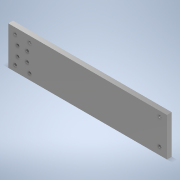
# Autodesk Inventor part: Corner Stands
Saved by Autodesk Inventor 2020 (Build 240168000, 168)
## iProperties
Created: 2020-03-17
Part Number: Corner Stands
Material: Generic
Document SubType Name: Modeling
Designer: DasNick
Density: 1 g/cm^3
Appearance: Anodized - Light Gray
Author: DasNick
Autodesk Inventor part; units mm, degrees
ref_plane "YZ Plane" through (0, 0, 0) normal (1, 0, 0) x (0, 1, 0)
ref_plane "XZ Plane" through (0, 0, 0) normal (0, 1, 0) x (-1, 0, 0)
ref_plane "XY Plane" through (0, 0, 0) normal (0, 0, 1) x (1, 0, 0)
sketch "Sketch1" plane through (0, 0, 0) normal (0, 0, 1) x (1, 0, 0)
  line L0 (246.3741, 31.7234) -> (246.3741, -882.6766) construction
  line L1 (234.1821, 31.7234) -> (231.3881, 31.7234) construction
  line L2 (223.2601, 31.7234) -> (220.4661, 31.7234) construction
  line L3 (199.5111, 31.7234) -> (196.0821, 31.7234) construction
  line L4 (182.3661, 31.7234) -> (178.9371, 31.7234) construction
  line L5 (246.3741, 31.7234) -> (170.1741, 31.7234)
  line L6 (170.1741, 31.7234) -> (170.1741, -69.8766)
  line L7 (170.1741, -69.8766) -> (246.3741, -69.8766)
  line L8 (246.3741, -69.8766) -> (246.3741, 31.7234)
  circle A0 centre (227.3241, 15.8484) radius 3.9688
  line L9 (208.2741, -69.8766) -> (208.2741, 31.7234) construction
  line L10 (246.3741, -19.0766) -> (170.1741, -19.0766) construction
  circle A1 centre (227.3241, -54.0016) radius 3.9688
  circle A2 centre (189.2241, 15.8484) radius 3.9688
  circle A3 centre (189.2241, -54.0016) radius 3.9688
  point P0 (0, 0)
  dimension "d0" = 76.2
  dimension "d1" = 101.6
  dimension "d2" = 7.9375
  dimension "d3" = 15.875
  dimension "d4" = 19.05
  constraints: 12 end point, 4 centre point, 4 midpoint, 3 symmetric about line, 2 parallel, 1 horizontal, 1 perpendicular, 3 other
  measures "d0" distance of L7.end L6.end
  measures "d1" distance of L6.end L5.end
  measures "d2" diameter of A0
  measures "d3" distance from line of L5 A0.centre
  measures "d4" distance from line of L0 A0.centre
extrude "Extrusion1" add sketch "Sketch1" along normal blind 12.7
sketch "Sketch3" plane through (0, 0, 0) normal (0, 0, -1) x (-1, 0, 0)
  line L0 (-186.0491, -41.3016) -> (-230.4991, -41.3016)
  line L1 (-230.4991, -41.3016) -> (-230.4991, 3.1484)
  line L2 (-230.4991, 3.1484) -> (-186.0491, 3.1484)
  line L3 (-186.0491, 3.1484) -> (-186.0491, -41.3016)
  line L4 (-170.1741, -69.8766) -> (-246.3741, -69.8766) projected
  line L5 (-170.1741, 31.7234) -> (-170.1741, -69.8766) projected
  line L6 (-246.3741, 31.7234) -> (-170.1741, 31.7234) projected
  circle A0 centre (-195.5741, -6.3766) radius 6.35
  circle A1 centre (-195.5741, -31.7766) radius 6.35
  circle A2 centre (-220.9741, -6.3766) radius 6.35
  circle A3 centre (-220.9741, -31.7766) radius 6.35
  point P0 (0, 0)
  dimension "d16" = 44.45
  dimension "d17" = 44.45
  dimension "d18" = 28.575
  dimension "d19" = 15.875
  dimension "d23" = 12.7
  dimension "d24" = 9.525
  dimension "d25" = 9.525
  dimension "d28" = 25.4
  dimension "d31" = 25.4
  constraints: 8 end point, 4 centre point, 2 horizontal, 2 parallel, 1 perpendicular, 1 vertical, 7 other
  measures "d16" distance of L0.end L1.end
  measures "d17" distance of L0.start L0.end
  measures "d18" distance between parallel lines of L4 L0
  measures "d19" distance between parallel lines of L5 L3
  measures "d23" diameter of A0
  measures "d24" distance from line of L2 A0.centre
  measures "d25" distance from line of L3 A0.centre
  measures "d28" distance of A0.centre A1.centre
  measures "d31" distance of A0.centre A2.centre
extrude "Extrusion3" cut sketch "Sketch3" against normal blind 7.9375 contours A0 | A1 | A2 | A3
sketch "Sketch4" plane through (195.5741, -6.3766, 7.9375) normal (0, 0, -1) x (-1, 0, 0)
  circle A0 centre (0, 0) radius 6.35 projected
  circle A1 centre (0, -25.4) radius 6.35 projected
  circle A2 centre (-25.4, 0) radius 6.35 projected
  circle A3 centre (-25.4, -25.4) radius 6.35 projected
  circle A4 centre (0, 0) radius 3.9688
  line L0 (0, 0) -> (0, -11.1628) construction
  line L1 (0, 0) -> (-15.7699, 0) construction
  circle A5 centre (0, -25.4) radius 3.9688
  circle A6 centre (-25.4, 0) radius 3.9688
  circle A7 centre (-25.4, -25.4) radius 3.9688
  point P0 (195.5741, 6.3766)
  dimension "d36" = 7.9375
  dimension "d37" = 7.9375
  dimension "d38" = 7.9375
  dimension "d39" = 7.9375
  constraints: 4 centre point, 4 coincident, 4 end point, 1 horizontal, 1 vertical
  measures "d36" diameter of A4
  measures "d37" diameter of A5
  measures "d38" diameter of A6
  measures "d39" diameter of A7
extrude "Extrusion4" cut sketch "Sketch4" against normal blind 7.9375 contours A4 | A5 | A6 | A7
sketch "Sketch5" plane through (0, 0, 12.7) normal (0, 0, 1) x (1, 0, 0)
  line L0 (589.2741, -69.8766) -> (589.2741, 844.5234)
  line L1 (246.3741, -69.8766) -> (589.2741, -69.8766)
  line L2 (246.3741, 31.7234) -> (170.1741, 31.7234) projected
  line L3 (246.3741, 31.7234) -> (589.2741, 31.7234)
  line L4 (376.7143, 0.5706) -> (376.7143, -56.5544)
  line L5 (376.7143, 18.2956) -> (376.7143, 9.7706)
  line L6 (376.7143, 18.2956) -> (376.7143, 23.7956)
  line L7 (376.7143, -62.0544) -> (376.7143, -56.5544)
  circle A0 centre (227.3241, 15.8484) radius 3.9688 projected
  circle A1 centre (227.3241, -54.0016) radius 3.9688 projected
  circle A2 centre (570.2241, 18.2956) radius 3.9688
  circle A3 centre (570.2241, -50.0328) radius 3.9688
  line L8 (246.3741, 31.7234) -> (246.3741, -69.8766)
  point P0 (0, 0)
  dimension "d42" = 7.9375
  dimension "d43" = 7.9375
  dimension "d44" = 19.05
  dimension "d45" = 19.05
  constraints: 16 end point, 6 vertical, 2 centre point, 1 horizontal, 1 perpendicular, 1 point on line, 8 other
  measures "d42" diameter of A2
  measures "d43" diameter of A3
  measures "d44" distance from line of L0 A3.centre
  measures "d45" distance from line of L0 A2.centre
extrude "Extrusion5" add sketch "Sketch5" against normal blind 12.7 contours L1 L8 L3 L0
body "Solid1"
